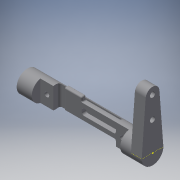
# Autodesk Inventor part: SR-T-07
Saved by Autodesk Inventor 2019.4 (Build 234330000, 330)
## iProperties
Created: 2019-06-15
Part Number: SR-T-07
Material: 一般
Document SubType Name: Modeling
Designer: Koki Shinjo
Mass: 0.441219 g
Surface Area: 7.10788 cm^2
Volume: 0.441219 cm^3
Density: 1 g/cm^3
Appearance: 既定
Author: Koki Shinjo
Autodesk Inventor part; units mm, degrees
ref_plane "YZ Plane" through (0, 0, 0) normal (1, 0, 0) x (0, 1, 0)
sketch "スケッチ1" plane through (0, 0, 0) normal (0, 0, 1) x (1, 0, 0)
  line L0 (0, 0) -> (0, 2.5)
  line L1 (0, 2.5) -> (-29, 2.5)
  line L2 (-29, 2.5) -> (-29, 0)
  line L3 (-29, 0) -> (0, 0)
  dimension "d0" = 29
  dimension "d1" = 2.5
  constraints: 8 end point, 3 perpendicular, 1 vertical
  measures "d0" distance of L0.end L1.end
  measures "d1" distance of L0.start L0.end
revolve "回転1" add sketch "スケッチ1" angle 360 about axis through (-29, 0, 0) along (1, 0, 0)
sketch "スケッチ2" plane through (0, 0, 0) normal (1, 0, 0) x (0, 0, -1)
  circle A0 centre (0, 6.7) radius 0.6
  circle A1 centre (0, 11.7) radius 0.6
  circle A2 centre (0, 11.7) radius 1.6
  line L0 (-1.5953, 11.8231) -> (-2.4926, 0.1923)
  circle A3 centre (0, 0) radius 2.5 projected
  line L1 (2.4926, 0.1923) -> (1.5953, 11.8231)
  dimension "d3" = 1.2
  dimension "d4" = 5
  dimension "d5" = 6.7
  dimension "d6" = 3.2
  constraints: 4 end point, 4 point on circle, 4 tangent, 3 centre point, 2 vertical alignment, 1 coincident, 1 equal radius
  measures "d3" diameter of A1
  measures "d4" distance of A1.centre A0.centre
  measures "d5" distance of point (0, 0) A0.centre
  measures "d6" diameter of A2
extrude "押し出し1" add sketch "スケッチ2" against normal blind 2.5 contours A2 | A2 L1 A3 L0
ref_plane "作業平面1" through (0, 0, 0) normal (0, 1, 0) x (-1, 0, 0)
sketch "スケッチ3" plane through (0, 0, 0) normal (0, 1, 0) x (-1, 0, 0)
  line L0 (0, 1.5953) -> (0, 2.4926) construction
  line L1 (0, 1.5953) -> (2.5, 1.5953) construction
  line L2 (2.5, 2.4926) -> (2.5, 1.5953) construction
  line L3 (2.5, 2.4926) -> (0, 2.4926) construction
  line L4 (0, 0.6) -> (2.5, 0.6) construction
  line L5 (0, 1.5953) -> (0, -1.5953) construction
  line L6 (0, -2.4926) -> (0, -1.5953) construction
  point P0 (0, 0)
sketch "スケッチ4" plane through (0, 0, 0) normal (0, 0, 1) x (1, 0, 0)
  line L0 (-15.9, 0) -> (-15.9, 3.5)
  line L1 (-15.9, 3.5) -> (-19.999, 3.5)
  line L2 (-19.999, 3.5) -> (-19.999, 0)
  line L3 (-15.9, 0) -> (-19.999, 0)
  line L4 (-14.9, 4) -> (-14.9, -4) construction
  line L5 (-20.999, 4) -> (-20.999, -4) construction
  line L6 (-29, 2.5) -> (-2.5, 2.5) construction
  line L7 (-30.1038, 0) -> (-4.0505, 0) construction
  ellipse E0 centre (-16.5, 0) end of major axis (-16.5, -4) minor radius 0 construction
  ellipse E1 centre (-19.399, 0) end of major axis (-19.399, 4) minor radius 0 construction
  point P0 (0, 0)
  dimension "d37" = 1
  dimension "d38" = 1
  dimension "d39" = 1
  constraints: 10 end point, 2 horizontal, 1 parallel, 1 point on line, 4 other
  measures "d37" distance between parallel lines of L6 L1
  measures "d38" distance between parallel lines of L5 L2
  measures "d39" distance between parallel lines of L4 L0
extrude "押し出し2" add sketch "スケッチ4" along normal mid plane 1
fillet "フィレット1" radius 0.5 2 edges at (-19.999, 3.5, 0) (-15.9, 3.5, 0)
fillet "フィレット2" radius 0.5 2 edges at (-15.9, 2.4873, -0.2513) (-15.9, 2.4873, 0.2513)
sketch "スケッチ5" plane through (-19.499, 3.5, -0.5) normal (0, 1, 0) x (1, 0, 0)
  line L0 (0, -1) -> (-0.5, -1) projected
  line L1 (-0.5, -1) -> (11.5, -1)
  line L2 (11.5, -1) -> (11.5, 0) construction
  line L3 (11.5, 0) -> (-0.5, 0)
  line L4 (-0.5, 0) -> (-0.5, -1)
  line L5 (-0.5, 0) -> (0, 0) projected
  line L6 (12, -1.5) -> (-1, -1.5)
  line L7 (-1, -1.5) -> (-1, 0.5)
  line L8 (-1, 0.5) -> (12, 0.5)
  line L9 (12, 0.5) -> (12, -1.5) construction
  line L10 (11.5, -1) -> (11.5, -1.5)
  line L11 (11.5, 0) -> (11.5, 0.5)
  point P0 (19.499, -0.5)
  dimension "d18" = 12
  dimension "d19" = 0.5
  constraints: 20 end point, 4 parallel, 4 point on line, 3 perpendicular, 1 horizontal, 3 other
  measures "d18" distance of L2.end L3.end
  measures "d19" distance between parallel lines of L1 L6
extrude "押し出し3" cut sketch "スケッチ5" against normal up to next
ref_plane "作業平面2" through (0, 0, 0) normal (0, 0, 1) x (1, 0, 0)
sketch "スケッチ6" plane through (0, 0, 0) normal (0, 0, 1) x (1, 0, 0)
  line L0 (-7.999, 2.4495) -> (-15.4, 2.4495) construction
  line L1 (-15.4, 2.4495) -> (-15.4, 2.4495) construction
  line L2 (-15.4, 2.4495) -> (-7.999, 2.4495) construction
  line L3 (-7.999, 2.4495) -> (-7.999, 2.2913) construction
  line L4 (-7.999, 2.2913) -> (-20.499, 2.2913) construction
  line L5 (-20.499, 2.2913) -> (-20.499, 2.2913) construction
  line L6 (-20.499, 2.2913) -> (-7.999, 2.2913) construction
  line L7 (-7.999, 2.2913) -> (-7.999, 2.4495) construction
  line L8 (-19.999, -2.4495) -> (-19.999, -2.4495) construction
  line L9 (-19.999, -2.4495) -> (-7.999, -2.4495) construction
  line L10 (-7.999, -2.4495) -> (-7.999, -2.2913) construction
  line L11 (-7.999, -2.2913) -> (-20.499, -2.2913) construction
  line L12 (-20.499, -2.2913) -> (-20.499, -2.2913) construction
  line L13 (-20.499, -2.2913) -> (-7.999, -2.2913) construction
  line L14 (-7.999, -2.2913) -> (-7.999, -2.4495) construction
  line L15 (-7.999, -2.4495) -> (-19.999, -2.4495) construction
  line L16 (-2.5, 0.1923) -> (0, 0.1923) construction
  line L17 (-2.5, 0.1923) -> (-2.5, 0.1923) construction
  line L18 (-2.5, 0.1923) -> (0, 0.1923) construction
  line L19 (0, 0.1923) -> (0, 0.1923) construction
  line L20 (-29, -2.5) -> (-29, 2.5) construction
  line L21 (-7.999, -2.4495) -> (-19.999, -2.4495) construction
  line L22 (-7.999, 2.4495) -> (-7.999, -2.4495) construction
  line L23 (-15.4, 2.4495) -> (-7.999, 2.4495) construction
  line L24 (-15.9, 2.958) -> (-15.9, 3) construction
  arc A0 (-15.9, 3) -> (-16.4, 3.5) centre (-16.4, 3) ccw construction
  line L25 (-16.4, 3.5) -> (-19.499, 3.5) construction
  arc A1 (-19.499, 3.5) -> (-19.999, 3) centre (-19.499, 3) ccw construction
  line L26 (-19.999, 3) -> (-19.999, -2.4495) construction
  line L27 (-19.999, -2.5) -> (-19.999, -2.4495) projected
  line L28 (-19.999, -2.5) -> (-7.999, -2.5)
  line L29 (-7.999, -2.5) -> (-7.999, -1)
  line L30 (-7.999, -1) -> (-19.999, -1)
  line L31 (-19.999, -1) -> (-19.999, -2.5)
  line L32 (-7.999, 1.5) -> (-15.9, 1.5)
  line L33 (-15.9, 1.5) -> (-15.9, 0)
  line L34 (-15.9, 0) -> (-7.999, 0)
  line L35 (-7.999, 0) -> (-7.999, 1.5)
  line L36 (-29, 2.5) -> (-2.5, 2.5) construction
  point P0 (0, 0)
  dimension "d22" = 1.5
  dimension "d23" = 1
  dimension "d24" = 1
  constraints: 16 end point, 4 parallel, 3 point on line, 2 horizontal, 2 perpendicular, 1 other
  measures "d22" distance between parallel lines of L28 L30
  measures "d23" distance between parallel lines of L32 L36
  measures "d24" distance between parallel lines of L30 L34
extrude "押し出し4" cut sketch "スケッチ6" along normal mid plane 1
fillet "フィレット3" radius 0.5 6 edges at (-7.999, 0, 0) (-7.999, 1.5, 0) (-7.999, -1, 0) (-15.9, 0, 0) (-15.9, 1.5, 0) (-19.999, -1, 0)
move faces "移動1" translate (-2, 0, 0) faces at (-20.499, 0.8022, 0.4409)
delete faces "削除1" heal yes whole lump no faces at (-16.15, 3.433, 0.1667) (-19.5364, 3.4986, 0.1667)
fillet "フィレット4" radius 0.3 2 edges at (-17.9495, 3.5, 0.5) (-17.9495, 3.5, -0.5)
delete faces "削除2" heal yes whole lump no faces at (-15.8985, 2.9397, -0.352)
delete faces "削除3" heal yes whole lump no faces at (-19.932, -0.75, 0.1667)
delete faces "削除4" heal yes whole lump no faces at (-8.0859, -1.2183, 0.1667)
fillet "フィレット5" radius 0.3 10 edges at (-15.9, 3.4121, -0.4121) (-15.9, 2.8247, -0.5) (-15.9, 3.4121, 0.4121) (-15.9, 2.8247, 0.5) (-15.9, 3.5, 0) (-19.999, 1.1, 0.5) (-19.999, 3.5, 0) (-19.999, 3.4121, -0.4121) (-19.999, 1.1, -0.5) (-19.999, 3.4121, 0.4121)
fillet "フィレット6" radius 0.3 4 edges at (-15.9896, 2.4655, 0.4138) (-15.9896, 2.4655, -0.4138) (-15.9, 2.498, -0.1001) (-15.9, 2.498, 0.1001)
fillet "フィレット7" radius 0.3 1 edges at (-7.999, -1, 0)
delete faces "削除5" heal yes whole lump no faces at (-12.8323, 0.7638, 1)
fillet "フィレット8" radius 0.5 1 edges at (-22.499, 0, -1)
sketch "スケッチ7" plane through (-15.4, 0, 0.5) normal (0, 0, 1) x (1, 0, 0)
  line L0 (7.401, 2.4495) -> (7.401, -2.2913) construction
  line L1 (7.401, -2.2913) -> (-6.599, -2.2913) construction
  line L2 (-7.099, -2.4495) -> (-7.099, 2.4495) construction
  line L3 (-6.599, 2.2913) -> (7.401, 2.2913) construction
  line L4 (7.401, 2.2913) -> (7.401, 2.4495) construction
  line L5 (7.401, 2.4495) -> (-0.32, 2.4495) construction
  line L6 (-0.2, 2.4936) -> (-0.2, 2.4936) construction
  line L7 (-0.32, 2.4495) -> (7.401, 2.4495) construction
  line L8 (12.9, 0.1923) -> (15.4, 0.1923) construction
  line L9 (12.9, 0.1923) -> (12.9, 0.1923) construction
  line L10 (12.9, 0.1923) -> (15.4, 0.1923) construction
  line L11 (15.4, 0.1923) -> (15.4, 0.1923) construction
  line L12 (-13.6, -2.5) -> (-13.6, 2.5) construction
  line L13 (-13.6, 2.5) -> (12.9, 2.5) projected
  line L14 (-10.099, 2.5) -> (10.401, 2.5)
  line L15 (10.401, 2.5) -> (10.401, -2.5)
  line L16 (10.401, -2.5) -> (-10.099, -2.5)
  line L17 (-10.099, -2.5) -> (-10.099, 2.5)
  point P0 (15.4, 0)
  dimension "d40" = 3
  dimension "d41" = 3
  constraints: 8 end point, 2 parallel, 1 horizontal, 1 horizontal alignment, 1 perpendicular, 1 point on line, 4 other
  measures "d40" distance between parallel lines of L17 L2
  measures "d41" distance between parallel lines of L0 L15
extrude "押し出し5" cut sketch "スケッチ7" along normal up to next
sketch "スケッチ8" plane through (-15.4, 0, 0.5) normal (0, 0, 1) x (1, 0, 0)
  circle A0 centre (8.901, 0) radius 0.7 construction
  circle A1 centre (-8.599, 0) radius 0.7 construction
  circle A2 centre (-8.599, 0) radius 0.55
  circle A3 centre (8.901, 0) radius 0.55
  point P0 (15.4, 0)
  dimension "d44" = 1.1
  constraints: 2 centre point, 2 coincident, 1 equal radius
  measures "d44" diameter of A3
extrude "押し出し6" cut sketch "スケッチ8" against normal up to next
